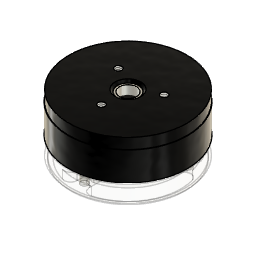
3_screw_R1_v7 (Autodesk Fusion 360 archive; units mm, degrees)
design "PTZ2204"
Autodesk Fusion 360 part; units mm, degrees
cylinder "CylinderPrimitive1" add diameter 27.75 height 4.5 placed x (1, 0, 0) y (0, 1, 0) z (0, 0, 1) at (0, 0, 0) makes body 1 in component "Stator"
sketch "Sketch2" plane through (0, 0, 0) normal (0, 0, -1) x (1, 0, 0) in component "Stator"
  circle A0 centre (0, 0) radius 13.875
  circle A1 centre (0, 0) radius 13.375
  circle A2 centre (0, 0) radius 5.5
  line L0 (-1.435, 5.8671) -> (-1.435, 12.3721)
  line L1 (0, 0) -> (0, 13.875) construction
  arc A3 (-1.435, 5.8671) -> (-5.8023, -1.6776) centre (0, 0) ccw
  arc A4 (-1.435, 12.3721) -> (-11.4373, -4.931) centre (0, 0) ccw
  line L2 (-5.8023, -1.6776) -> (-11.4373, -4.931)
  line L3 (0, 0) -> (-12.0161, -6.9375) construction
  line L4 (-4.3635, -4.1763) -> (-9.997, -7.4288)
  arc A5 (-4.3635, -4.1763) -> (4.354, -4.1862) centre (0, 0) ccw
  line L5 (4.354, -4.1862) -> (9.989, -7.4395)
  arc A6 (-9.997, -7.4288) -> (9.989, -7.4395) centre (0, 0) ccw
  line L6 (5.7985, -1.6908) -> (11.432, -4.9433)
  arc A7 (5.7985, -1.6908) -> (1.4483, 5.8638) centre (0, 0) ccw
  line L7 (1.4483, 5.8638) -> (1.4483, 12.3705)
  arc A8 (11.432, -4.9433) -> (1.4483, 12.3705) centre (0, 0) ccw
  circle A9 centre (0, 0) radius 4.75
  point P0 (0, 10.265)
  point P1 (-8.8898, -5.1325)
  point P2 (8.8898, -5.1325)
  dimension "d3" = -0.5
  dimension "d6" = 11
  dimension "d7" = 12.08
  dimension "d12" = 0.92
  dimension "d17" = 120
  dimension "d18" = 1.435
  dimension "d19" = 1.4483
  dimension "d21" = 360
  dimension "d26" = 9.5
  dimension "d126" = 17.7795
  constraint concentric A0 A2
  constraint concentric A2 A3
  constraint coincident A0.centre A1.centre
  constraint coincident A0 L1.end
  constraint vertical L1
  constraint coincident L1 P0
  constraint concentric A2 A4
  constraint coincident A0 L3.end
  constraint concentric A4 A9
  measures "d6" diameter of A2
  measures "d7" diameter of A3
  measures "d12" distance of A1 A4
  measures "d17" angle of L1 L3
  measures "d18" distance of L0 L1
  measures "d19" distance of L2 L3
  measures "d26" diameter of A9
  measures "d126" distance of P0 P1
extrude "Extrude1" cut sketch "Sketch2" against normal blind 0.6 contours A0 bodies 1 in component "Stator"
extrude "Extrude2" cut sketch "Sketch2" against normal blind 2 contours L0 A3 A4 L2 | L4 A5 L5 A6 | L6 A7 L7 A8 bodies 1 in component "Stator"
fillet "Fillet1" radius 1.5 12 edges at (-9.997, 7.4288, 1) (-11.4373, 4.931, 1) (-4.3635, 4.1763, 1) (-5.8023, 1.6776, 1) (-1.435, -5.8671, 1) (1.4483, -5.8638, 1) (5.7985, 1.6908, 1) (4.354, 4.1862, 1) (11.432, 4.9433, 1) (9.989, 7.4395, 1) (1.4483, -12.3705, 1) (-1.435, -12.3721, 1) on bodies 1 in component "Stator"
extrude "Extrude3" cut sketch "Sketch2" against normal up to surface (4.5 mm away) contours A9 bodies 1 in component "Stator"
extrude "Extrude4" cut sketch "Sketch2" against normal blind 0.7 contours A2 bodies 1 in component "Stator"
hole "Hole1" at (8.8898, 5.1325, 0) at (0, -10.265, 0) at (-8.8898, 5.1325, 0) direction (0, 0, 1) diameter 1.623 depth 6 tip angle 118 bodies 1 in component "Stator"
thread "Thread1" "ISO Metric profile 2.0 M2x0.4 6H" major diameter 2.074 minor diameter 1.623 pitch 0.4 angle 60 resizes the face on face at (-8.8493, 5.943, 1.5) on face at (0.0404, -9.4545, 1.5) on face at (8.9302, 5.943, 1.5) on bodies 1 in component "Stator"
cylinder "CylinderPrimitive1'" add diameter 27.93 height 9.55 placed x (1, 0, 0) y (0, 1, 0) z (0, 0, 1) at (0, 0, 4.5) separate body makes body 2 in component "Rotor"
extrude "Extrude1'" cut 1 faces at (1.7745, 2.6223, 4.5) along direction (0, 0, 1) blind 0.36 on bodies 2 bodies 2 in component "Rotor"
sketch "Sketch2 (2)" plane through (0, 0, 14.05) normal (0, 0, 1) x (-1, 0, 0) in component "Rotor"
  circle A0 centre (0, 0) radius 13.965
  circle A1 centre (0, 0) radius 2
  circle A2 centre (0, 0) radius 2.5
  circle A3 centre (0, 0) radius 13.865
  line L0 (0, 0) -> (0, 13.965) construction
  point P0 (0, 6.2354)
  point P1 (-5.4, -3.1177)
  point P2 (5.4, -3.1177)
  dimension "d40" = 4
  dimension "d41" = 5
  dimension "d42" = -0.1
  dimension "d46" = 360
  dimension "d127" = 10.8
  constraint concentric A0 A1
  constraint concentric A1 A2
  constraint coincident A0.centre A1.centre
  constraint coincident A0 L0.end
  constraint vertical L0
  constraint coincident L0 P0
  measures "d40" diameter of A1
  measures "d41" diameter of A2
  measures "d127" distance of P0 P1
extrude "Extrude2'" cut sketch "Sketch2 (2)" against normal blind 2.5 contours A0 bodies 2 in component "Rotor"
extrude "Extrude3'" cut sketch "Sketch2 (2)" against normal through all contours A1 | A2 bodies 2 in component "Rotor"
chamfer "Chamfer2" distance 0.5 angle 45 1 edges at (2.3308, -0.904, 14.05) on bodies 2 in component "Rotor"
hole "Hole1'" at (-5.4, 3.1177, 14.05) at (5.4, 3.1177, 14.05) at (0, -6.2354, 14.05) direction (0, 0, -1) diameter 1.623 depth 6 tip angle 180 bodies 2 in component "Rotor"
thread "Thread1'" "ISO Metric profile 2.0 M2x0.4 6H" major diameter 2.074 minor diameter 1.623 pitch 0.4 angle 60 resizes the face on face at (-5.3192, 2.3102, 10.05) on face at (0.0808, -7.0429, 10.05) on face at (5.4808, 2.3102, 10.05) on bodies 2 in component "Rotor"
sketch "Sketch3" plane through (0, 0, 4.86) normal (0, 0, -1) x (1, 0, 0) in component "Rotor"
  circle A0 centre (0, 0) radius 2.5
  circle A1 centre (0, 0) radius 13.965
  circle A2 centre (0, 0) radius 13.215
  dimension "d72" = 0.75
  constraint coincident A0.centre A1.centre
  measures "d72" distance of A1 A2
extrude "Extrude6" cut sketch "Sketch3" against normal blind 8.35 contours A2 bodies 2 in component "Rotor"
sketch "Sketch4" plane through (0, 0, 13.21) normal (0, 0, -1) x (1, 0, 0) in component "Rotor"
  circle A0 centre (5.4, -3.1177) radius 0.8115
  circle A1 centre (-5.4, -3.1177) radius 0.8115
  circle A2 centre (0, 6.2354) radius 0.8115
  circle A3 centre (0, 0) radius 2.5
  circle A4 centre (0, 0) radius 13.215
  circle A5 centre (0, 0) radius 7.1244
  dimension "d128" = 14.2489
  constraint concentric A3 A5
  measures "d128" diameter of A5
extrude "Extrude7" add sketch "Sketch4" along normal blind 1.65 contours A5 bodies 2 in component "Rotor"
chamfer "Chamfer3" distance 1.6 angle 45 1 edges at (-6.6423, -2.5763, 13.21) on bodies 2 in component "Rotor"
sketch "Sketch5" plane through (0, 0, 11.56) normal (0, 0, -1) x (1, 0, 0) in component "Rotor"
  circle A0 centre (0, 0) radius 3.4
  line L0 (0, -3.4) -> (0, -7.1244) construction
  line L1 (0.47, -3.3674) -> (0.47, -5.2622)
  line L2 (0.47, -5.2622) -> (-0.47, -5.2622)
  line L3 (-0.47, -5.2622) -> (-0.47, -3.3674)
  line L4 (0, -3.4) -> (0, 0) construction
  circle A1 centre (0, 0) radius 7.1244
  circle A2 centre (5.4, -3.1177) radius 0.8115
  circle A3 centre (-5.4, -3.1177) radius 0.8115
  circle A4 centre (0, 6.2354) radius 0.8115
  circle A5 centre (0, 0) radius 2.5
  dimension "d80" = 6.8
  dimension "d81" = 0.94
  constraint coincident A0.centre L4.end
  constraint coincident L0.end A1
  constraint vertical L0
  constraint coincident A0 L1.start
  constraint parallel L0 L1
  constraint perpendicular L0 L2
  constraint coincident A0 L3.end
  constraint perpendicular L2 L3
  constraint symmetric L0 L1 L3
  constraint coincident A0 L0.start
  constraint midpoint L0 L2
  constraint vertical L4
  measures "d80" diameter of A0
  measures "d81" distance of L1.end L2.end
extrude "Extrude8" add sketch "Sketch5" along normal blind 1.65 contours A0 | A0 L1 L2 L3 | A5 bodies 2 in component "Rotor"
fillet "Fillet1'" radius 0.4 2 edges at (0.47, 3.3674, 10.735) (-0.47, 3.3674, 10.735) on bodies 2 in component "Rotor"
extrude "Extrude5" add sketch "Sketch2 (2)" against normal blind 15.28 from surface at -0.5 separate body contours A2 makes body 3 in component "Rotor"
sketch "Sketch6" plane through (0, 0, -1.73) normal (0, 0, -1) x (1, 0, 0) in component "Rotor"
  circle A0 centre (0, 0) radius 2
  circle A1 centre (0, 0) radius 2.5
  circle A2 centre (0, 0) radius 2.25
  dimension "d86" = 4.5
  constraint coincident A0.centre A1.centre
  measures "d86" diameter of A2
extrude "Extrude9" cut sketch "Sketch6" against normal blind 0.5 from surface at -1.65 contours A1 bodies 3 in component "Rotor"
chamfer "Chamfer4" distance 0.25 angle 45 1 edges at (-12.3207, -4.7787, 4.86) on bodies 2 in component "Rotor"
sketch "Sketch7" plane through (0, 0, 4.86) normal (0, 0, -1) x (1, 0, 0) in component "Rotor"
  circle A0 centre (0, 0) radius 13.965
  circle A1 centre (0, 0) radius 13.465
  circle A2 centre (0, 0) radius 13.215
  circle A3 centre (0, 0) radius 11.215
  line L0 (-2, -11.0352) -> (-2, -13.0628)
  line L1 (2, -11.0352) -> (2, -13.0628)
  line L2 (0, 0) -> (0, -0.2539) construction
  line L3 (0, -0.2539) -> (0, -13.215) construction
  dimension "d91" = 2
  dimension "d92" = 4
  constraint concentric A2 A3
  constraint coincident A2 L0.end
  constraint coincident A2 L1.end
  constraint parallel L0 L1
  constraint coincident A3 L0.start
  constraint coincident A3 L1.start
  constraint coincident A0.centre A1.centre
  constraint vertical L2
  constraint coincident A2 L3.end
  constraint parallel L2 L3
  constraint symmetric L0 L1 L3
  measures "d91" distance of A2 A3
  measures "d92" distance of L0 L1
extrude "Extrude10" add sketch "Sketch7" against normal blind 4 from surface at -0.25 separate body contours A2 A3 L0 L1 picked at (1.5566, -11.7643) makes body 4 in component "Rotor"
fillet "Fillet2" radius 0.15 4 faces at (1.5589, 11.1061, 7.7767) (1.5566, 11.7643, 5.11) (-2, 11.7111, 6.4433) (2, 11.7111, 6.4433) on bodies 4 in component "Rotor"
pattern_circular "C-Pattern1" count 14 over 360 about axis through (0, 0, 13.55) along (0, 0, -1) of bodies 4 makes body 5 at (7.0058, 11.2052, 6.5433) makes body 6 at (11.1737, 7.0558, 6.5433) makes body 7 at (13.1286, 1.509, 6.5433) makes body 8 at (13.1286, -1.509, 6.5433) makes body 9 at (9.3653, -9.3235, 6.5433) makes body 10 at (7.0058, -11.2052, 6.5433) makes body 11 at (1.4502, -13.1352, 6.5433) makes body 12 at (-7.0058, -11.2052, 6.5433) makes body 13 at (-9.3653, -9.3235, 6.5433) makes body 14 at (-12.4831, -4.3367, 6.5433) makes body 15 at (-12.4831, 4.3367, 6.5433) makes body 16 at (-9.3653, 9.3235, 6.5433) makes body 17 at (-4.3925, 12.4636, 6.5433) in component "Rotor"
sketch "Sketch3 (2)" plane through (0, 0, 4.5) normal (0, 0, 1) x (-1, 0, 0) in component "Stator"
  circle A0 centre (0, 10.265) radius 0.8115
  circle A1 centre (-8.8898, -5.1325) radius 0.8115
  circle A2 centre (8.8898, -5.1325) radius 0.8115
  circle A3 centre (0, 0) radius 4.75
  circle A4 centre (0, 0) radius 13.875
  circle A5 centre (0, 0) radius 12.455
  dimension "d63" = 24.91
  constraint concentric A3 A5
  measures "d63" diameter of A5
extrude "Extrude5'" cut sketch "Sketch3 (2)" against normal up to surface (2.5 mm away) contours A5 bodies 1 in component "Stator"
sketch "Sketch4 (2)" plane through (0, 0, 2) normal (0, 0, 1) x (-1, 0, 0) in component "Stator"
  circle A0 centre (0, 0) radius 4.75
  circle A1 centre (8.8898, -5.1325) radius 0.8115
  circle A2 centre (-8.8898, -5.1325) radius 0.8115
  circle A3 centre (0, 10.265) radius 0.8115
  arc A4 (8.7236, -8.8897) -> (8.423, -6.52) centre (7.673, -7.819) ccw
  arc A5 (8.7236, -8.8897) -> (12.0644, -3.0948) centre (0, 0) ccw
  arc A6 (9.8614, -4.0211) -> (12.0644, -3.0948) centre (10.6114, -2.7221) ccw
  line L0 (9.8614, -4.0211) -> (6.7341, -2.2156)
  arc A7 (5.9952, -0.7342) -> (6.7341, -2.2156) centre (7.4841, -0.9165) ccw
  arc A8 (5.9952, -0.7342) -> (2.3511, 5.5636) centre (0, 0) ccw
  arc A9 (1.435, 6.9453) -> (2.3511, 5.5636) centre (2.935, 6.9453) ccw
  line L1 (1.435, 6.9453) -> (1.435, 10.5545)
  arc A10 (3.3369, 11.9997) -> (1.435, 10.5545) centre (2.935, 10.5545) ccw
  arc A11 (3.3369, 11.9997) -> (-3.352, 11.9955) centre (0, 0) ccw
  arc A12 (-1.4483, 10.5508) -> (-3.352, 11.9955) centre (-2.9483, 10.5508) ccw
  line L2 (-1.4483, 10.5508) -> (-1.4483, 6.9397)
  arc A13 (-2.3618, 5.5591) -> (-1.4483, 6.9397) centre (-2.9483, 6.9397) ccw
  arc A14 (-2.3618, 5.5591) -> (-5.9938, -0.7457) centre (0, 0) ccw
  arc A15 (-6.7323, -2.2299) -> (-5.9938, -0.7457) centre (-7.4823, -0.9309) ccw
  line L3 (-6.7323, -2.2299) -> (-9.858, -4.0345)
  arc A16 (-12.0605, -3.11) -> (-9.858, -4.0345) centre (-10.608, -2.7355) ccw
  arc A17 (-12.0605, -3.11) -> (-8.7124, -8.9006) centre (0, 0) ccw
  arc A18 (-8.4131, -6.5297) -> (-8.7124, -8.9006) centre (-7.6631, -7.8287) ccw
  line L4 (-8.4131, -6.5297) -> (-5.2858, -4.7241)
  arc A19 (-3.6334, -4.8249) -> (-5.2858, -4.7241) centre (-4.5358, -6.0231) ccw
  arc A20 (-3.6334, -4.8249) -> (3.6427, -4.8179) centre (0, 0) ccw
  arc A21 (5.2973, -4.7154) -> (3.6427, -4.8179) centre (4.5473, -6.0144) ccw
  line L5 (5.2973, -4.7154) -> (8.423, -6.52)
  circle A22 centre (0, 0) radius 4.5
  circle A23 centre (0, 0) radius 4
  circle A24 centre (0, 0) radius 5.5
  dimension "d64" = 9
  dimension "d65" = 8
  dimension "d66" = 11
  constraint concentric A0 A22
  constraint concentric A22 A23
  constraint concentric A22 A24
  measures "d64" diameter of A22
  measures "d65" diameter of A23
  measures "d66" diameter of A24
extrude "Extrude6'" add sketch "Sketch4 (2)" along normal blind 3 contours A0 | A24 bodies 1 in component "Stator"
extrude "Extrude7'" add sketch "Sketch4 (2)" along normal blind 6 from surface at 2 contours A22 bodies 1 in component "Stator"
sketch "Sketch5 (2)" plane through (0, 0, 10) normal (0, 0, 1) x (-1, 0, 0) in component "Stator"
  circle A0 centre (0, 0) radius 4
  circle A1 centre (0, 0) radius 4.5
  line L0 (1.725, 1.7428) -> (-1.725, 1.7428)
  line L1 (-1.725, 1.7428) -> (-1.725, 5.5339)
  line L2 (-1.725, 5.5339) -> (1.725, 5.5339)
  line L3 (1.725, 5.5339) -> (1.725, 1.7428)
  line L4 (0, 0) -> (0, 5.5339) construction
  dimension "d100" = 3.45
  constraint horizontal L0
  constraint vertical L1
  constraint horizontal L2
  constraint vertical L3
  constraint coincident A0.centre A1.centre
  constraint midpoint L2 L4.end
  constraint vertical L4
  measures "d100" distance of L1 L3
extrude "Extrude8'" add sketch "Sketch5 (2)" along normal blind 0.9 contours A0 A1 L1 L3 picked at (-1.5405, 3.8633) bodies 1 in component "Stator"
ref_plane "WorkPlane1" through (-0.002, -2.0146, 2) normal (0, 0, 1) x (1, 0, 0) in component "Stator"
sketch "Sketch7 (2)" plane through (0, 0, 2) normal (0, 0, 1) x (1, 0, 0) in component "Stator"
  circle A0 centre (0, 0) radius 11.4
  circle A1 centre (-8.8898, 5.1325) radius 0.8115
  circle A2 centre (8.8898, 5.1325) radius 0.8115
  circle A3 centre (0, -10.265) radius 0.8115
  arc A4 (1.75, -11.2649) -> (-1.75, -11.2649) centre (0, -11.2045) ccw
  line L0 (0, -10.265) -> (0, -14.2869) construction
  arc A5 (8.8807, 7.148) -> (10.6307, 4.1169) centre (9.7034, 5.6023) ccw
  arc A6 (-10.6307, 4.1169) -> (-8.8807, 7.148) centre (-9.7034, 5.6023) ccw
  circle A7 centre (0, 0) radius 5.5
  circle A8 centre (0, 0) radius 5.5
  dimension "d104" = 22.8
  dimension "d105" = 3.5
  dimension "d107" = 360
  constraint coincident A0.centre A7.centre
  constraint tangent A3 A4
  constraint coincident A0 A4.start
  constraint coincident A0 A4.end
  constraint coincident A3.centre L0.start
  constraint vertical L0
  constraint symmetric A4.end A4.start L0
  measures "d104" diameter of A0
  measures "d105" distance of A4.end A4.start
extrude "Extrude9'" add sketch "Sketch7 (2)" along normal blind 1.6 separate body contours A0 A4 A5 A6 makes body 18 in component "Stator"
fillet "Fillet2'" radius 1.25 6 edges at (-8.8807, 7.148, 2.8) (-10.6307, 4.1169, 2.8) (1.75, -11.2649, 2.8) (-1.75, -11.2649, 2.8) (8.8807, 7.148, 2.8) (10.6307, 4.1169, 2.8) on bodies 18 in component "Stator"
sketch "Sketch1" plane through (0, 0, 5) normal (0, 0, 1) x (-1, 0, 0) in component "Stator"
  circle A0 centre (0, 0) radius 4.5
  circle A1 centre (0, 0) radius 5.5
  circle A2 centre (0, 0) radius 11
  line L0 (0, 0) -> (2.15, 10.7878)
  line L1 (0, 0) -> (-2.15, 10.7878)
  line L2 (0, 0) -> (0, 11) construction
  circle A3 centre (0, 0) radius 9.6834
  circle A4 centre (0, 0) radius 6
  line L3 (-0.5, 5.9791) -> (-0.5, 9.6705)
  line L4 (0.5, 5.9791) -> (0.5, 9.6705)
  dimension "d112" = 22
  dimension "d113" = 4.3
  dimension "d114" = 12
  dimension "d123" = 1
  dimension "d125" = 1.3166
  constraint coincident A0.centre A1.centre
  constraint coincident A2 L0.end
  constraint coincident A2 L1.end
  constraint coincident A2 L2.end
  constraint vertical L2
  constraint symmetric L0 L1 L2
  constraint concentric A3 A4
  constraint coincident A4 L3.start
  constraint coincident A3 L3.end
  constraint coincident A3 L4.end
  constraint parallel L3 L4
  constraint coincident A4 L4.start
  measures "d112" diameter of A2
  measures "d113" distance of L0.end L1.end
  measures "d114" diameter of A4
  measures "d123" distance of L3 L4
  measures "d125" distance of A2 A3
extrude "Extrude10'" add sketch "Sketch1" along normal blind 4.3 separate body contours A0 A1 L0 L1 | A0 A1 L0 L1 | A1 L0 L1 A4 | A1 L0 L1 A4 makes body 19 in component "Stator"
extrude "Extrude11" add sketch "Sketch1" along normal up to surface (4.3 mm away) contours A2 L0 L1 A3 | A3 A4 L3 L4 picked at (0.0556, 10.5449) bodies 19 in component "Stator"
pattern_circular "C-Pattern1'" count 12 over 360 about axis through (0, 0, 1.75) along (0, 0, 1) of bodies 19 makes body 20 at (4.0757, -7.3926, 5) makes body 21 at (7.226, -4.3644, 5) makes body 22 at (8.4401, -0.1667, 5) makes body 23 at (6.327, 3.4605, 9.3) makes body 24 at (4.3644, 7.226, 5) makes body 25 at (0.1667, 8.4401, 5) makes body 26 at (-4.0757, 7.3926, 5) makes body 27 at (-7.226, 4.3644, 5) makes body 28 at (-8.4401, 0.1667, 5) makes body 29 at (-7.3926, -4.0757, 5) makes body 30 at (-4.3644, -7.226, 9.3) in component "Stator"
combine "Combine1" operation add target body 19 tool bodies 23 22 21 20 26 28 30 27 24 25 29 in component "Stator"
component "Stator" placed x (1, 0, 0) y (0, 1, 0) z (0, 0, 1) at (0, 0, 0)
component "Rotor" placed x (1, 0, 0) y (0, 1, 0) z (0, 0, 1) at (0, 0, 0)
equation "d57 = -15.78 mm + 0.5 mm"
equation "d63 = ( 12.455 * 2 ) * 1 mm"
equation "d76 = 8.15 mm - 6.5 mm"
named bodies: "Stator", "Rotor", "Shaft", "Magnet", "Magnet1 (1)", "Magnet1 (2)", "Magnet1 (3)", "Magnet1 (4)", "Magnet1 (5)", "Magnet1 (6)", "Magnet1 (7)", "Magnet1 (8)", "Magnet1 (9)", "Magnet1 (10)", "Magnet1 (11)", "Magnet1 (12)", "Magnet1 (13)", "PCB", "Winding Frame", "Winding Frame (1)", "Winding Frame (2)", "Winding Frame (3)", "Winding Frame (4)", "Winding Frame (5)", "Winding Frame (6)", "Winding Frame (7)", "Winding Frame (8)", "Winding Frame (9)", "Winding Frame (10)", "Winding Frame (11)"
